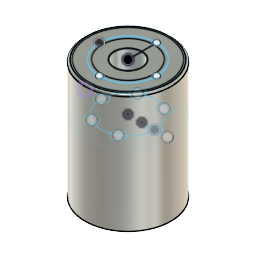
End Effector v16 (Autodesk Fusion 360 design; units mm, degrees)
Autodesk Fusion 360 part; units mm, degrees
sketch "Sketch1" plane through (0, 0, 0) normal (0, 0, 1) x (1, 0, 0)
  circle A0 centre (0, 0) radius 10.85
  dimension "d1" = 21.7
  constraint coincident A0.centre origin
  measures "d1" diameter of A0
extrude "Extrude1" add sketch "Sketch1" along normal blind 12
sketch "Sketch2" plane through (0, 0, 12) normal (0, 0, 1) x (-1, 0, 0)
  circle A0 centre (0, 0) radius 10.85
  line L0 (0, 0) -> (0, -6.5)
  circle A1 centre (0, 0) radius 6.5
  circle A2 centre (0, 0) radius 9.95
  circle A3 centre (0, 0) radius 3.5
  circle A4 centre (7.25, 0) radius 0.75
  circle A5 centre (0, 0) radius 7.25
  circle A6 centre (0, 7.25) radius 0.75
  circle A7 centre (-7.25, 0) radius 0.75
  circle A8 centre (0, -7.25) radius 0.75
  dimension "d6" = 6.5
  dimension "d7" = 19.9
  dimension "d8" = 7
  dimension "d13" = 1.5
  dimension "d15" = 360
  constraint coincident A0.centre L0.start
  constraint vertical L0
  constraint coincident L0.end A1
  constraint concentric A1 A2
  constraint concentric A1 A5
  constraint coincident A4.centre A5
  measures "d6" distance of A0.centre L0.end
  measures "d7" diameter of A2
  measures "d8" diameter of A3
  measures "d13" diameter of A4
extrude "Extrude2" cut sketch "Sketch2" against normal up to surface (12 mm away) contours A3
extrude "Extrude4" cut sketch "Sketch2" against normal blind 2.5 contours A5 A7 | A5 A8 | A5 A6 | A5 A7 | A4 A5 | A5 A8 | A5 A6 | A4 A5
sketch "Sketch5" plane through (0, 0, 0) normal (0, 0, -1) x (1, 0, 0)
  circle A0 centre (0, 0) radius 3.5
  circle A1 centre (0, 0) radius 10.85
  line L0 (3.5, 0) -> (9.95, 0)
  circle A2 centre (0, 0) radius 6.725
  circle A3 centre (6.725, 0) radius 1.5
  circle A4 centre (3.3625, 5.824) radius 1.5
  circle A5 centre (-3.3625, 5.824) radius 1.5
  circle A6 centre (-6.725, 0) radius 1.5
  circle A7 centre (-3.3625, -5.824) radius 1.5
  circle A8 centre (3.3625, -5.824) radius 1.5
  point P0 (3.5, 0)
  point P1 (-10.85, 0)
  dimension "d40" = 3
  dimension "d42" = 360
  dimension "d49" = 13.45
  constraint coincident P0 L0.start
  constraint coincident A0.centre A1.centre
  constraint midpoint L0 A3.centre
  measures "d40" diameter of A3
  measures "d49" distance of A3.centre A6.centre
extrude "Extrude8" cut sketch "Sketch5" against normal blind 5 contours L0 A2 A3 | L0 A2 A3 | L0 A2 A3 | L0 A2 A3 | A2 A4 | A2 A4 | A2 A8 | A2 A8 | A2 A5 | A2 A5 | A2 A7 | A2 A7 | A2 A6 | A2 A6
extrude "Extrude9" add 1 faces at (0.2703, -8.0526, 0) along direction (0, 0, -1) blind 1.3
sketch "Sketch8" plane through (0, 0, 0) normal (0, 1, 0) x (1, 0, 0)
extrude "Extrude10" add 1 faces at (0.2703, -8.0526, -1.3) along direction (0, 0, -1) blind 16.7
extrude "Extrude11" add sketch "Sketch5" along normal blind 10 contours L0 A2 A3 | L0 A2 A3 | L0 A2 A3 | L0 A2 A3 | A2 A4 | A2 A4 | A2 A8 | A2 A8 | A2 A5 | A2 A5 | A2 A7 | A2 A7 | A2 A6 | A2 A6
fillet "Fillet7" radius 0.5 1 edges at (-10.1158, -3.9235, 12)
